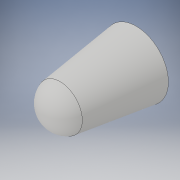
# Autodesk Inventor part: pawn2
Saved by Autodesk Inventor 2019 (Build 230136000, 136)
## iProperties
Created: 2018-11-27
Part Number: pawn2
Material: Generic
Document SubType Name: Modeling
Designer: Solomon Kritz
Density: 1 g/cm^3
Appearance: Default
Author: Solomon Kritz
Autodesk Inventor part; units mm, degrees
ref_plane "YZ Plane" through (0, 0, 0) normal (1, 0, 0) x (0, 1, 0)
ref_plane "XZ Plane" through (0, 0, 0) normal (0, 1, 0) x (-1, 0, 0)
ref_plane "XY Plane" through (0, 0, 0) normal (0, 0, 1) x (1, 0, 0)
sketch "Sketch3" plane through (0, 0, 0) normal (0, 1, 0) x (-1, 0, 0)
  line L0 (0, 0) -> (-10.5, 0)
  line L1 (0, 0) -> (0, 30)
  line L2 (-10.5, 0) -> (-7.2665, 24.7713)
  arc A0 (0, 30) -> (-7.2665, 24.7713) centre (-0.1825, 22.59) ccw
  dimension "d0" = 10.5
  dimension "d1" = 30
  constraints: 6 end point, 2 point on circle, 1 centre point, 1 horizontal, 1 vertical
  measures "d0" distance of L0.start L0.end
  measures "d1" distance of L0.start L1.end
revolve "Revolution1" add sketch "Sketch3" angle 360 about axis through (0, 0, 0) along (0, 0, 1)
body "Solid1"
